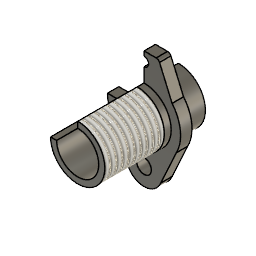
Bearing Brass (Autodesk Fusion 360 design; units mm, degrees)
Autodesk Fusion 360 part; units mm, degrees
note: some values were not read from the file. Set by a fixed rule: which face or edge a step refers to.
sketch "Sketch2" plane through (0, 0, 0) normal (0, 1, 0) x (1, 0, 0)
  circle A0 centre (0, 0) radius 15.875
  dimension "d1" = 31.75
  constraint coincident A0.centre origin
  measures "d1" diameter of A0
extrude "Extrude1" add sketch "Sketch2" along normal blind 41.275 thin wall 1.27 inside makes body 1
thread "Thread1" "ANSI Unified Screw Threads 1.5 1 1/2-6 UNC 1 1/2-6 UNC 1A" major diameter 37.6936 minor diameter 32.9997 pitch 4.2333 angle 60 resizes the face on face at (15.7961, 27.5167, 1.5806) on bodies 1
sketch "Sketch3" plane through (0, 41.275, 0) normal (0, 1, 0) x (-1, 0, 0)
  circle A0 centre (0, 0) radius 18.8468
  circle A1 centre (0, 0) radius 19.05
  circle A2 centre (0, 0) radius 14.605
  dimension "d6" = 38.1
  constraint coincident A0.centre A1.centre
  measures "d6" diameter of A1
extrude "Extrude2" add sketch "Sketch3" along normal blind 28.575 thin wall 1.778 inside separate body contours A0 | A2 makes body 2
sketch "Sketch4" plane through (0, 0, 0) normal (0, 1, 0) x (1, 0, 0)
  circle A0 centre (0, 0) radius 19.05
  line L0 (0, -19.05) -> (0, 2.54)
  line L1 (0, -19.05) -> (0, 0)
  line L2 (19.05, 0) -> (0, 0)
  arc A1 (0, -19.05) -> (19.05, 0) centre (0, 0) ccw
  line L3 (0, 0) -> (0, -19.05)
  line L4 (0, 0) -> (-19.05, 0)
  arc A2 (-19.05, 0) -> (0, -19.05) centre (0, 0) ccw
  dimension "d11" = 38.1
  constraint coincident A0.centre L1.end
  constraint coincident A0 L0.start
  constraint vertical L0
  constraint parallel L0 L1
  constraint coincident A0 L2.start
  constraint perpendicular L1 L2
  constraint coincident A0 L4.end
  constraint perpendicular L1 L4
  measures "d11" diameter of A0
extrude "Extrude3" cut sketch "Sketch4" along normal blind 69.85 contours A0 L0 L1 L3 L4 A2 bodies 1 2
ref_plane "WorkPlane1" through (0, 46.0375, 0) normal (0, -1, 0) x (1, 0, 0)
sketch "Sketch5" plane through (0, 46.0375, 0) normal (0, -1, 0) x (-1, 0, 0)
  circle A0 centre (0, 0) radius 25.4
  line L0 (0, -25.4) -> (0, -38.1)
  line L1 (0, -38.1) -> (-8.4403, -38.1)
  line L2 (-10.774, -36.5628) -> (-25.2318, -2.9181)
  arc A1 (-10.774, -36.5628) -> (-8.4403, -38.1) centre (-8.4403, -35.56) ccw
  line L3 (25.4, 0) -> (11.6135, 35.5182)
  line L4 (-25.4, 0) -> (-11.6221, 35.5215)
  line L5 (-25.4, 0) -> (-63.5, 0) construction
  arc A2 (11.6135, 35.5182) -> (-11.6221, 35.5215) centre (-0.0049, 31.0085) ccw
  circle A3 centre (0, -31.75) radius 3.175
  line L6 (0, 0) -> (0, -25.4)
  line L7 (0, 0) -> (25.4, 0)
  line L8 (0, 0) -> (25.4, 0)
  arc A4 (0, -25.4) -> (25.4, 0) centre (0, 0) ccw
  dimension "d15" = 50.8
  dimension "d16" = 2.54
  dimension "d17" = 38.1
  dimension "d18" = 111.2
  dimension "d19" = 38.1
  dimension "d20" = 6.35
  constraint coincident A0.centre L6.start
  constraint coincident A0 L0.start
  constraint vertical L0
  constraint perpendicular L0 L1
  constraint coincident A0 L2.end
  constraint tangent L1 A1
  constraint tangent L2 A1
  constraint coincident A0 L3.start
  constraint horizontal L5
  constraint coincident A0 L4.start
  constraint tangent L3 A2
  constraint midpoint L0 A3.centre
  constraint parallel L0 L6
  constraint perpendicular L6 L7
  constraint coincident L6 A0.centre
  measures "d15" diameter of A0
  measures "d16" radius of A1
  measures "d17" distance of L3.start L3.end
  measures "d18" angle of L4 L5
  measures "d19" distance of L4.start L4.end
  measures "d20" diameter of A3
extrude "Extrude4" add sketch "Sketch5" against normal blind 7.9375 contours A0 L2 L3 L4 L6 L7 L8 | A0 L4 | A0 L2 | A0 L3 L4 A2 | A0 L0 L1 L2 A1 A3 | A0 L3 bodies 2
sketch "Sketch6" plane through (0, 46.0375, 0) normal (0, -1, 0) x (1, 0, 0)
  arc A0 (-17.0688, 0) -> (0, 17.0688) centre (0, 0) ccw
  line L0 (0, 17.0688) -> (0, 0)
  line L1 (0, 0) -> (-17.0688, 0)
  circle A1 centre (0, 0) radius 15.24
  constraint coincident A0.centre L0.end
extrude "Extrude5" cut sketch "Sketch6" 1 faces at (-11.3176, 46.0375, -0.8348) against normal blind 17.78 contours L0 L1 A1 picked at (-6.0731, 8.1128) on bodies 2 bodies 2
hole "Hole1" at (0.0049, 46.0375, -31.0085) direction (0, 1, 0) diameter 10.16 depth 12.7 tip angle 118 bodies 2
sketch "Sketch7" plane through (0, 46.0375, 0) normal (0, -1, 0) x (1, 0, 0)
  circle A0 centre (0.0049, -31.0085) radius 5.08
  arc A1 (-18.8468, 0) -> (0, 18.8468) centre (0, 0) ccw
  line L0 (-18.8468, 0) -> (-25.4, 0)
  arc A2 (-25.4, 0) -> (-18.7485, -17.1363) centre (0, 0) ccw
  line L1 (-18.7485, -17.1363) -> (-11.6135, -35.5182)
  arc A3 (-11.6135, -35.5182) -> (11.6221, -35.5215) centre (0.0049, -31.0085) ccw
  line L2 (11.6221, -35.5215) -> (18.7568, -17.1273)
  arc A4 (18.7568, -17.1273) -> (19.4828, 16.2967) centre (0, 0) ccw
  line L3 (19.4828, 16.2967) -> (10.774, 36.5628)
  arc A5 (10.774, 36.5628) -> (8.4403, 38.1) centre (8.4403, 35.56) ccw
  line L4 (8.4403, 38.1) -> (0, 38.1)
  line L5 (0, 38.1) -> (0, 34.925)
  arc A6 (0, 28.575) -> (0, 34.925) centre (0, 31.75) ccw
  line L6 (0, 28.575) -> (0, 18.8468)
  line L7 (-23.6788, -9.191) -> (-11.6135, -35.5182)
  line L8 (23.6788, -9.191) -> (11.6221, -35.5215)
  constraint midpoint A2 L7.start
  constraint coincident L1.end A3.start
  constraint coincident A4 L8.start
  constraint coincident A3.end L2.start
extrude "Extrude6" add sketch "Sketch7" against normal blind 7.9375 contours A2 L1 L7 | L2 A4 L8 bodies 2
equation "d1 = ( 5 / 4 ) * 1 in"
equation "d2 = ( 13 / 8 ) * 1 in"
equation "d8 = ( 9 / 8 ) * 1 in"
equation "d12 = 11 / 4 * 1 in"
equation "d14 = -( 44 / 16 - 15 / 16 - 26 / 16 ) * 1 in"
equation "d15 = 1,5 in + 0,50 in"
equation "d21 = -5 / 16 * 1 in"
equation "d28 = -5 / 16 * 1 in"
